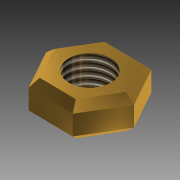
# Autodesk Inventor part: Nut
Saved by Autodesk Inventor 2015 (Build 190159000, 159)
## iProperties
Created: 2015-06-22
Part Number: Nut
Material: 真鍮
Document SubType Name: Modeling
Designer: kenta
Density: 8.49 g/cm^3
Appearance: 真鍮 - つや出し
Mass: 0.351778 g
Surface Area: 0.947248 cm^2
Volume: 0.0414344 cm^3
Author: kenta
Autodesk Inventor part; units mm, degrees
ref_plane "YZ Plane" through (0, 0, 0) normal (1, 0, 0) x (0, 1, 0)
ref_plane "XZ Plane" through (0, 0, 0) normal (0, 1, 0) x (-1, 0, 0)
ref_plane "XY Plane" through (0, 0, 0) normal (0, 0, 1) x (1, 0, 0)
sketch "スケッチ1" plane through (0, 0, 0) normal (0, 0, 1) x (1, 0, 0)
  line L0 (1.5437, -2.775) -> (-1.6314, -2.7243)
  line L1 (-1.6314, -2.7243) -> (-3.175, 0.0506)
  line L2 (-3.175, 0.0506) -> (-1.5437, 2.775)
  line L3 (-1.5437, 2.775) -> (1.6314, 2.7243)
  line L4 (1.6314, 2.7243) -> (3.175, -0.0506)
  line L5 (3.175, -0.0506) -> (1.5437, -2.775)
  point P0 (0, 0)
  point P1 (0, 0)
  dimension "d0" = 5.5
  constraints: 12 end point, 1 coincident, 13 other
  measures "d0" distance between parallel lines of L4 L1
extrude "押し出し1" add sketch "スケッチ1" along normal blind 2.4
sketch "スケッチ2" plane through (0, 0, 2.4) normal (0, 0, 1) x (1, 0, 0)
  circle A0 centre (0, 0) radius 1.5
  dimension "d3" = 3
  constraints: 1 centre point, 1 coincident
  measures "d3" diameter of A0
extrude "押し出し2" cut sketch "スケッチ2" against normal blind 2.4
thread "ねじ1" size "M3x0.5" class "6H" standard "ANSI Metric M Profile" full length
chamfer "面取り1" distance 0.5 angle 45 12 edges at (2.3593, -1.4128, 2.4) (2.4032, 1.3369, 2.4) (0.0438, 2.7497, 2.4) (-2.3593, 1.4128, 2.4) (-2.4032, -1.3369, 2.4) (-0.0438, -2.7497, 2.4) (-0.0438, -2.7497, 0) (2.3593, -1.4128, 0) (2.4032, 1.3369, 0) (0.0438, 2.7497, 0) (-2.3593, 1.4128, 0) (-2.4032, -1.3369, 0)
